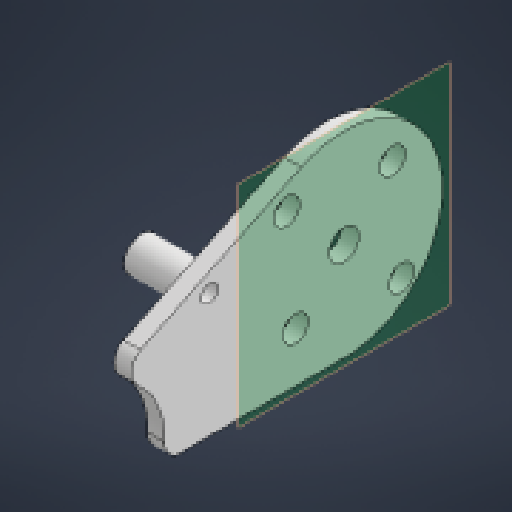
# Autodesk Inventor part: Motor_Cover
Saved by Autodesk Inventor 2024.2 (Build 282272000, 272)
## iProperties
Created: 2024-02-26
Part Number: Motor_Cover
Material: 一般
Document SubType Name: Modeling
Designer: Hanaoka
Density: 1 g/cm^3
Appearance: 既定
Author: Hanaoka
Autodesk Inventor part; units mm, degrees
ref_plane "YZ Plane" through (0, 0, 0) normal (1, 0, 0) x (0, 1, 0)
ref_plane "XZ Plane" through (0, 0, 0) normal (0, 1, 0) x (-1, 0, 0)
ref_plane "XY Plane" through (0, 0, 0) normal (0, 0, 1) x (1, 0, 0)
ref_plane "作業平面1" through (-52.2521, -19.4961, 18.3784) normal (-1, 0, 0) x (0, 0, 1)
sketch "スケッチ1" plane through (-52.2521, -19.4961, 18.3784) normal (-1, 0, 0) x (0, 0, 1)
  line L0 (27.6413, -15.0569) -> (18.8577, -11.6363) projected
  arc A0 (27.6413, -15.0569) -> (32.8377, -3.1521) centre (30, -9) ccw projected
  line L1 (5.0205, 10.3462) -> (32.8377, -3.1521) projected
  arc A1 (5.0205, 10.3462) -> (0, -11.5) centre (0, 0) ccw projected
  line L2 (18.1319, -11.5) -> (0, -11.5) projected
  arc A2 (18.8577, -11.6363) -> (18.1319, -11.5) centre (18.1319, -13.5) ccw projected
  circle A3 centre (0, 0) radius 1.75 projected
  circle A4 centre (30, -9) radius 3.6 projected
  arc A5 (27.2373, -0.4345) -> (21.8406, -12.798) centre (30, -9) ccw
  circle A6 centre (6.7175, 6.7175) radius 1.6 projected
  circle A7 centre (-5.6569, 5.6569) radius 1.6 projected
  circle A8 centre (-6.7175, -6.7175) radius 1.6 projected
  circle A9 centre (5.6569, -5.6569) radius 1.6 projected
  circle A10 centre (15.7301, 2.9263) radius 2
  circle A11 centre (15.7301, 2.9263) radius 1 projected
  circle A12 centre (-5.6569, 5.6569) radius 1.5
  circle A13 centre (6.7175, 6.7175) radius 1.5
  circle A14 centre (5.6569, -5.6569) radius 1.5
  circle A15 centre (-6.7175, -6.7175) radius 1.5
  point P0 (-18.3784, 19.4961)
  dimension "d0" = 9
  dimension "d4" = 4
  dimension "d8" = 3
  constraints: 6 centre point, 5 coincident, 3 equal radius, 2 point on circle, 2 point on line
  measures "d0" radius of A5
  measures "d4" diameter of A10
  measures "d8" diameter of A15
extrude "押し出し1" add sketch "スケッチ1" along normal blind 2 contours A10 | L0 A2 L2 A1 L1 A5 | A6 | A7 | A8 | A9
fillet "フィレット1" radius 2 2 edges at (-53.2521, -19.9306, 45.6157) (-53.2521, -32.2941, 40.2191)
sketch "スケッチ2" plane through (-52.2521, -19.4961, 18.3784) normal (1, 0, 0) x (0, 0, -1)
  circle A0 centre (-15.7301, 2.9263) radius 2
  circle A1 centre (-15.7301, 2.9263) radius 1 projected
  point P0 (18.3784, 19.4961)
  dimension "d5" = 4
  constraints: 1 centre point, 1 concentric
  measures "d5" diameter of A0
extrude "押し出し2" add sketch "スケッチ2" against normal blind 8
